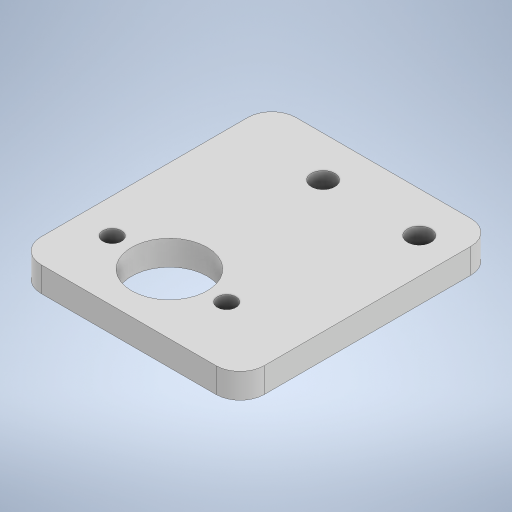
# Autodesk Inventor part: soporte eje z
Saved by Autodesk Inventor 2024.2 (Build 282272000, 272)
## iProperties
Created: 2023-12-16
Part Number: soporte eje z
Material: Genérico
Document SubType Name: Modeling
Designer: sergi
Density: 1 g/cm^3
Appearance: Valor por defecto
Author: sergi
Autodesk Inventor part; units mm, degrees
ref_plane "YZ Plane" through (0, 0, 0) normal (1, 0, 0) x (0, 1, 0)
ref_plane "XZ Plane" through (0, 0, 0) normal (0, 1, 0) x (-1, 0, 0)
ref_plane "XY Plane" through (0, 0, 0) normal (0, 0, 1) x (1, 0, 0)
sketch "Boceto1" plane through (0, 0, 0) normal (0, 1, 0) x (-1, 0, 0)
  line L0 (-23.2, -26.5) -> (23.2, -26.5)
  line L1 (23.2, -26.5) -> (23.2, 26.5)
  line L2 (23.2, 26.5) -> (-23.2, 26.5)
  line L3 (-23.2, 26.5) -> (-23.2, -26.5)
  line L4 (-23.2, -26.5) -> (23.2, 26.5) construction
  line L5 (23.2, -26.5) -> (-23.2, 26.5) construction
  line L6 (23.2, 26.5) -> (23.2, 21.8)
  line L7 (23.2, 21.8) -> (-23.2, 21.8)
  line L8 (23.2, 21.8) -> (11.9, 21.8)
  line L9 (11.9, 21.8) -> (11.9, 0)
  circle A0 centre (4.05, 13.95) radius 7.85
  line L10 (11.9, 13.95) -> (14, 13.95)
  line L11 (14, 13.95) -> (15.95, 13.95)
  circle A1 centre (15.95, 13.95) radius 1.95
  line L12 (-3.8, 13.95) -> (-5.9, 13.95)
  line L13 (-5.9, 13.95) -> (-7.85, 13.95)
  circle A2 centre (-7.85, 13.95) radius 1.95
  line L14 (23.2, -26.5) -> (23.2, -20.5)
  line L15 (23.2, -20.5) -> (-23.2, -20.5)
  line L16 (23.2, -20.5) -> (6.55, -20.5)
  line L17 (6.55, -20.5) -> (1.65, -20.5)
  line L18 (4.1, -20.5) -> (4.1, -18.05)
  circle A3 centre (4.1, -18.05) radius 2.45
  line L19 (1.65, -18.05) -> (-13.45, -18.05)
  line L20 (-13.45, -18.05) -> (-15.9, -18.05)
  circle A4 centre (-15.9, -18.05) radius 2.45
  point P0 (0, 0)
  point P1 (4.05, 21.8)
  dimension "d0" = 46.4
  dimension "d1" = 53
  dimension "d2" = 4.7
  dimension "d3" = 11.3
  dimension "d4" = 15.7
  dimension "d5" = 2.1
  dimension "d6" = 1.95
  dimension "d7" = 2.1
  dimension "d8" = 1.95
  dimension "d9" = 6
  dimension "d10" = 16.65
  dimension "d11" = 4.9
  dimension "d12" = 2.45
  dimension "d13" = 15.1
  dimension "d14" = 2.45
  constraints: 42 end point, 10 point on line, 4 coincident, 4 horizontal, 4 perpendicular, 3 horizontal alignment, 3 midpoint, 2 parallel, 2 point on circle, 2 tangent, 2 vertical, 1 centre point, 1 vertical alignment, 8 other
  measures "d0" distance of L2.end L1.end
  measures "d1" distance of L1.end L0.end
  measures "d2" distance of L1.end L6.end
  measures "d3" distance of L6.end L8.end
  measures "d4" diameter of A0
  measures "d5" distance of L10.start L10.end
  measures "d6" distance of L10.end L11.end
  measures "d7" distance of L12.start L12.end
  measures "d8" distance of L12.end L13.end
  measures "d9" distance of L0.end L14.end
  measures "d10" distance of L14.end L16.end
  measures "d11" distance of L16.end L17.end
  measures "d12" distance of L18.start L18.end
  measures "d13" distance of L19.start L19.end
  measures "d14" distance of L19.end L20.end
extrude "Extrusión1" add sketch "Boceto1" along normal blind 5.2 contours L3 L15 L1 L0 | L3 L7 A0 L9 L1 L15 A3 L19 A4 | L3 L2 L1 L7 | A4 L19 A3 L15 | L7 L9 A0
fillet "Empalme1" radius 5 4 edges at (-23.2, 2.6, 26.5) (-23.2, 2.6, -26.5) (23.2, 2.6, -26.5) (23.2, 2.6, 26.5)
